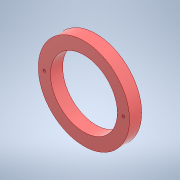
# Autodesk Inventor part: THz Polarizer
Saved by Autodesk Inventor 2020 (Build 240168000, 168)
## iProperties
Created: 2024-01-28
Part Number: THz Polarizer
Material: Phenolic Resin
Document SubType Name: Modeling
Designer: Scott
Density: 1.38 g/cm^3
Appearance: Smooth - Red
Mass: 28.0934 g
Surface Area: 82.8124 cm^2
Volume: 20.3575 cm^3
Author: Scott
Autodesk Inventor part; units mm, degrees
ref_plane "YZ Plane" through (0, 0, 0) normal (1, 0, 0) x (0, 1, 0)
ref_plane "XZ Plane" through (0, 0, 0) normal (0, 1, 0) x (-1, 0, 0)
ref_plane "XY Plane" through (0, 0, 0) normal (0, 0, 1) x (1, 0, 0)
sketch "Sketch1" plane through (0, 0, 0) normal (0, 0, 1) x (1, 0, 0)
  circle A0 centre (0, 0) radius 37.5
  circle A1 centre (0, 0) radius 32.5
  circle A2 centre (-32.5, 0) radius 1
  circle A3 centre (32.5, 0) radius 1
  circle A4 centre (0, 0) radius 27.5
  dimension "d0" = 75
  dimension "d1" = 65
  dimension "d2" = 2
  dimension "d3" = 2
  dimension "d4" = 55
  constraints: 5 centre point, 3 coincident, 2 point on circle
  measures "d0" diameter of A0
  measures "d1" diameter of A1
  measures "d2" diameter of A2
  measures "d3" diameter of A3
  measures "d4" diameter of A4
extrude "Extrusion1" add sketch "Sketch1" along normal blind 10 contours A0 | A3 A1 A2
body "Solid1"
